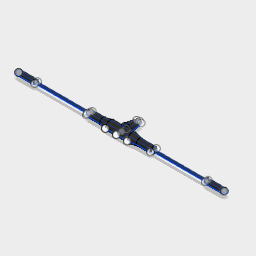
ImmortalTAntenna (Autodesk Fusion 360 design; units mm, degrees)
Autodesk Fusion 360 part; units mm, degrees
sketch "Sketch1" plane through (0, 0, 0) normal (0, 1, 0) x (1, 0, 0)
  line L0 (7.5, -3.5) -> (0, -3.5)
  line L1 (3.5, 3.5) -> (7.5, 3.5)
  line L2 (7.5, 3.5) -> (12.5, 2.5)
  line L3 (7.5, -3.5) -> (12.5, -2.5)
  line L4 (12.5, 2.5) -> (22, 2.5)
  line L5 (12.5, -2.5) -> (22, -2.5)
  line L6 (22.5, 2) -> (22.5, -2)
  line L7 (57.5, -1) -> (22.5, -1)
  line L8 (22.5, 1) -> (57.5, 1)
  line L9 (57.5, 1) -> (57.5, -1)
  line L10 (70.5, -2) -> (58.5, -2)
  line L11 (58.5, 2) -> (70.5, 2)
  line L12 (72.5, 0) -> (72.5, 0) construction
  line L13 (57.5, 1) -> (57.5, 1) construction
  line L14 (57.5, -1) -> (57.5, -1) construction
  arc A0 (58.5, 2) -> (57.5, 1) centre (58.5, 1) ccw
  arc A1 (57.5, -1) -> (58.5, -2) centre (58.5, -1) ccw
  arc A2 (72.5, 0) -> (70.5, 2) centre (70.5, 0) ccw
  arc A3 (70.5, -2) -> (72.5, 0) centre (70.5, 0) ccw
  line L15 (1.5764, 12.5) -> (0, 12.5)
  line L16 (3.5, 3.5) -> (2.0696, 12.0822)
  arc A4 (22.5, 2) -> (22, 2.5) centre (22, 2) ccw
  arc A5 (22, -2.5) -> (22.5, -2) centre (22, -2) ccw
  line L17 (-7.5, -3.5) -> (-12.5, -2.5)
  line L18 (-12.5, -2.5) -> (-22, -2.5)
  arc A6 (-22.5, -2) -> (-22, -2.5) centre (-22, -2) ccw
  line L19 (-22.5, 2) -> (-22.5, -2)
  arc A7 (-22, 2.5) -> (-22.5, 2) centre (-22, 2) ccw
  line L20 (-12.5, 2.5) -> (-22, 2.5)
  line L21 (-7.5, 3.5) -> (-12.5, 2.5)
  line L22 (-3.5, 3.5) -> (-7.5, 3.5)
  line L23 (-1.5764, 12.5) -> (0, 12.5)
  line L24 (-3.5, 3.5) -> (-2.0696, 12.0822)
  line L25 (-7.5, -3.5) -> (0, -3.5)
  line L26 (-22.5, 1) -> (-57.5, 1)
  line L27 (-57.5, -1) -> (-22.5, -1)
  arc A8 (-57.5, 1) -> (-58.5, 2) centre (-58.5, 1) ccw
  arc A9 (-70.5, 2) -> (-72.5, 0) centre (-70.5, 0) ccw
  arc A10 (-72.5, 0) -> (-70.5, -2) centre (-70.5, 0) ccw
  line L28 (-70.5, -2) -> (-58.5, -2)
  arc A11 (-58.5, -2) -> (-57.5, -1) centre (-58.5, -1) ccw
  line L29 (-58.5, 2) -> (-70.5, 2)
  line L30 (-57.5, 1) -> (-57.5, -1)
  arc A12 (-1.5764, 12.5) -> (-2.0696, 12.0822) centre (-1.5764, 12) ccw
  arc A13 (2.0696, 12.0822) -> (1.5764, 12.5) centre (1.5764, 12) ccw
  line L31 (-3.5, 3.5) -> (3.5, 3.5)
  line L32 (-72.5, 0) -> (72.5, 0)
  line L33 (0, 12.5) -> (0, 3.5)
  point P0 (0, 3.5)
  dimension "d28" = 7
  dimension "d37" = 1
  dimension "d38" = 1
  dimension "d39" = 2
  dimension "d40" = 2
  dimension "d43" = 0.5
  dimension "d44" = 0.5
  dimension "d45" = 0.5
  dimension "d46" = 0.5
  measures "d28" distance of L1.end L0.start
  measures "d37" radius of A0
  measures "d38" radius of A1
  measures "d39" radius of A2
  measures "d40" radius of A3
  measures "d43" radius of A4
  measures "d44" radius of A5
  measures "d45" radius of A12
  measures "d46" radius of A13
revolve "Revolve2" add sketch "Sketch1" angle 360 about axis through (0, 0, -12.5) along (0, 0, 1) contours L15 L16 A13 L31 L33 makes body 1
revolve "Revolve1" add sketch "Sketch1" angle 360 about axis through (-72.5, 0, 0) along (1, 0, 0) separate body contours L1 L2 L4 L6 A4 L19 A7 L20 L21 L22 L31 L32 | L6 L8 L9 L32 | L19 L26 L30 L32 | L9 L11 A0 A2 L32 | A8 A9 L29 L30 L32 makes body 2
extrude "Extrude1" add 1 faces at (-0.8429, -2.1478, -3.5) along direction (0, 0, 1) blind 3.5 on bodies 1 bodies 1 2
